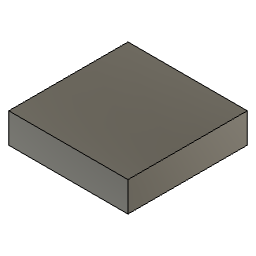
Square (Autodesk Fusion 360 design; units mm, degrees)
Autodesk Fusion 360 part; units mm, degrees
sketch "Square" plane through (0, 0, 0) normal (0, 0, 1) x (1, 0, 0)
  line L0 (12.7, -12.7) -> (0, -12.7)
  line L1 (0, -12.7) -> (0, 0)
  line L2 (12.7, 0) -> (12.7, -12.7)
  line L3 (0, 0) -> (12.7, 0)
extrude "Extrude1" add sketch "Square" along normal blind 3.175
